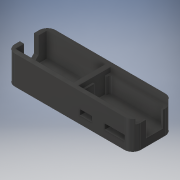
# Autodesk Inventor part: PiHolder
Saved by Autodesk Inventor 2019 (Build 230136000, 136)
## iProperties
Created: 2019-04-12
Part Number: PiHolder
Material: Generic
Document SubType Name: Modeling
Designer: Epsilon
Density: 1 g/cm^3
Appearance: Dark Gray
Author: Epsilon
Autodesk Inventor part; units mm, degrees
ref_plane "YZ Plane" through (0, 0, 0) normal (1, 0, 0) x (0, 1, 0)
ref_plane "XZ Plane" through (0, 0, 0) normal (0, 1, 0) x (-1, 0, 0)
ref_plane "XY Plane" through (0, 0, 0) normal (0, 0, 1) x (1, 0, 0)
sketch "Sketch2" plane through (0, 0, 0) normal (0, 1, 0) x (-1, 0, 0)
  line L0 (0, 0) -> (155, 0)
  line L1 (155, 0) -> (155, -50)
  line L2 (155, -50) -> (0, -50)
  line L3 (0, -50) -> (0, 0)
  dimension "d4" = 155
  dimension "d5" = 50
  constraints: 8 end point, 2 parallel, 1 horizontal, 1 perpendicular
  measures "d4" distance of L1.end L2.end
  measures "d5" distance of L0.end L1.end
extrude "Extrusion2" add sketch "Sketch2" along normal blind 35
sketch "Sketch4" plane through (0, 35, 0) normal (0, 1, 0) x (1, 0, 0)
  line L0 (0, 0) -> (0, 50) projected
  line L1 (0, 5) -> (-72, 5)
  line L2 (-72, 5) -> (-72, 45)
  line L3 (-72, 45) -> (0, 45)
  line L4 (0, 45) -> (0, 5)
  line L5 (-155, 50) -> (-155, 0) construction
  line L6 (-155, 25) -> (0, 25) construction
  dimension "d8" = 72
  dimension "d9" = 40
  constraints: 10 end point, 2 midpoint, 2 parallel, 2 perpendicular, 1 horizontal, 1 point on line, 1 other
  measures "d8" distance of L2.end L3.end
  measures "d9" distance of L1.end L2.end
extrude "Extrusion3" cut sketch "Sketch4" against normal blind 26
sketch "Sketch5" plane through (0, 9, 0) normal (0, 1, 0) x (1, 0, 0)
  line L0 (0, 5) -> (-72, 5) projected
  line L1 (-72, 45) -> (0, 45) projected
  line L2 (0, 5) -> (-72, 5)
  line L3 (-72, 5) -> (-72, 23)
  line L4 (-72, 45) -> (0, 45)
  line L5 (0, 45) -> (0, 16.68)
  line L6 (-2, 8) -> (-70, 8)
  line L7 (-70, 8) -> (-70, 23)
  line L8 (-70, 42) -> (-2, 42)
  line L9 (-2, 42) -> (-2, 37)
  line L10 (0, 50) -> (0, 0) construction
  line L11 (0, 25) -> (-72, 25) construction
  line L12 (-72, 5) -> (-72, 45) construction
  line L13 (-36, 5) -> (-36, 42) construction
  line L14 (0, 45) -> (0, 5) projected
  line L15 (-2, 16.68) -> (0, 16.68)
  line L16 (0, 37) -> (-2, 37)
  line L17 (-2, 16.68) -> (-2, 8)
  line L18 (0, 16.68) -> (0, 5)
  line L19 (-72, 5) -> (-72, 45) projected
  line L20 (-70, 38) -> (-72, 38)
  line L21 (-72, 38) -> (-72, 23) construction
  line L22 (-72, 23) -> (-70, 23)
  line L23 (-70, 23) -> (-70, 25) construction
  line L24 (-70, 38) -> (-70, 42)
  line L25 (-70, 23) -> (-70, 38) construction
  line L26 (-72, 23) -> (-72, 38)
  line L27 (-72, 38) -> (-72, 45)
  dimension "d12" = 68
  dimension "d13" = 34
  dimension "d17" = 20.32
  dimension "d43" = 15
  dimension "d44" = 4
  dimension "d52" = 8
  constraints: 44 end point, 17 parallel, 8 perpendicular, 4 horizontal, 4 midpoint, 3 point on line, 3 other
  measures "d12" distance of L8.start L8.end
  measures "d13" distance of L6.end L8.start
  measures "d17" distance of L16.start L5.end
  measures "d43" distance of L3.end L20.end
  measures "d44" distance between parallel lines of L8 L20
  measures "d52" distance between parallel lines of L1 L16
extrude "Extrusion5" add sketch "Sketch5" along normal blind 20 contours L0 L3 L22 L7 L6 L17 L15 L14 | L16 L9 L8 L24 L20 L19 L1 L5
fillet "Fillet2" radius 3 4 edges at (-2, 19, -8) (-70, 19, -8) (-70, 19, -42) (-2, 19, -42)
sketch "Sketch7" plane through (-155, 0, 0) normal (0, 0, 1) x (1, 0, 0)
  line L0 (89.9, 9) -> (104.9, 9)
  line L1 (104.9, 9) -> (104.9, 16)
  line L2 (104.9, 16) -> (89.9, 16)
  line L3 (89.9, 16) -> (89.9, 9)
  line L4 (89.9, 12.5) -> (104.9, 12.5) construction
  line L5 (97.4, 16) -> (97.4, 9) construction
  line L6 (88, 29) -> (88, 9) construction
  line L7 (88, 9) -> (150, 9) construction
  line L8 (85, 9) -> (85, 29) projected
  line L9 (120.4, 9) -> (132.4, 9)
  line L10 (132.4, 9) -> (132.4, 16) construction
  line L11 (132.4, 16) -> (120.4, 16)
  line L12 (120.4, 16) -> (120.4, 9)
  line L13 (133, 9) -> (145, 9)
  line L14 (145, 9) -> (145, 16)
  line L15 (145, 16) -> (133, 16)
  line L16 (133, 16) -> (133, 9) construction
  line L17 (126.4, 16) -> (126.4, 9) construction
  line L18 (139, 16) -> (139, 9) construction
  line L19 (132.4, 16) -> (133, 16) construction
  line L20 (132.4, 16) -> (133, 16)
  line L21 (132.4, 9) -> (133, 9)
  point P0 (155, 0)
  dimension "d29" = 15
  dimension "d30" = 7
  dimension "d32" = 0
  dimension "d35" = 12.4
  dimension "d36" = 12
  dimension "d37" = 7
  dimension "d38" = 12
  dimension "d39" = 7
  dimension "d40" = 41.4
  dimension "d41" = 54
  constraints: 38 end point, 8 midpoint, 6 parallel, 3 horizontal, 3 perpendicular, 2 point on line, 1 collinear
  measures "d29" distance of L2.end L1.end
  measures "d30" distance of L1.end L0.end
  measures "d32" distance between parallel lines of L7 L0
  measures "d35" distance between parallel lines of L8 L5
  measures "d36" distance of L11.end L10.end
  measures "d37" distance of L10.end L9.end
  measures "d38" distance of L15.end L14.end
  measures "d39" distance of L14.end L13.end
  measures "d40" distance between parallel lines of L8 L17
  measures "d41" distance between parallel lines of L8 L18
extrude "Extrusion7" cut sketch "Sketch7" against normal up to next
sketch "Sketch9" plane through (0, 35, 0) normal (0, 1, 0) x (1, 0, 0)
  line L0 (-78, 44.5) -> (-150, 44.5)
  line L1 (-150, 44.5) -> (-150, 33.89)
  line L2 (-150, 5.5) -> (-78, 5.5)
  line L3 (-78, 5.5) -> (-78, 44.5)
  line L4 (0, 50) -> (0, 0) construction
  line L5 (0, 25) -> (-155, 25) construction
  line L6 (-155, 0) -> (-155, 50) construction
  line L7 (-150, 25) -> (-78, 25) construction
  line L8 (-155, 50) -> (-155, 0) projected
  line L9 (-150, 16.11) -> (-155, 16.11)
  line L10 (-155, 16.11) -> (-155, 33.89)
  line L11 (-155, 33.89) -> (-150, 33.89)
  line L12 (-150, 33.89) -> (-150, 25) construction
  line L13 (-150, 25) -> (-155, 25) construction
  line L14 (-150, 33.89) -> (-150, 25) construction
  line L15 (-150, 16.11) -> (-150, 5.5)
  line L16 (-150, 25) -> (-150, 16.11) construction
  line L17 (-150, 25) -> (-150, 16.11) construction
  dimension "d45" = 72
  dimension "d46" = 39
  dimension "d47" = 5
  dimension "d50" = 17.78
  constraints: 30 end point, 8 parallel, 5 perpendicular, 4 midpoint, 2 collinear, 2 horizontal, 2 point on line
  measures "d45" distance between parallel lines of L3 L1
  measures "d46" distance between parallel lines of L2 L0
  measures "d47" distance between parallel lines of L6 L1
  measures "d50" distance between parallel lines of L9 L11
extrude "Extrusion8" cut sketch "Sketch9" against normal blind 30
fillet "Fillet3" radius 10 4 edges at (0, 17.5, 0) (0, 17.5, -50) (-155, 17.5, 0) (-155, 17.5, -50)
chamfer "Chamfer1" distance 8.89 angle 45 2 edges at (-152.5, 5, -33.89) (-152.5, 5, -16.11)
equation "\"d37\" = d30"
equation "\"d38\" = d36"
equation "\"d39\" = d37"
body "Solid2"
